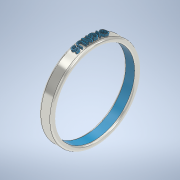
# Autodesk Inventor part: Repujado 3
Saved by Autodesk Inventor 2021 (Build 250183000, 183)
## iProperties
Created: 2021-01-13
Part Number: Repujado 3
Material: Genérico
Document SubType Name: Modeling
Designer: yosaf
Density: 1 g/cm^3
Appearance: Valor por defecto
Author: yosaf
Autodesk Inventor part; units mm, degrees
ref_plane "YZ Plane" through (0, 0, 0) normal (1, 0, 0) x (0, 1, 0)
ref_plane "XY Plane" through (0, 0, 0) normal (0, 0, 1) x (1, 0, 0)
sketch "Boceto1" plane through (0, 0, 0) normal (1, 0, 0) x (0, 1, 0)
  circle A0 centre (0, 0) radius 10
  dimension "d0" = 20
  constraints: 1 centre point, 1 coincident
  measures "d0" diameter of A0
extrude "Extrusión1" add sketch "Boceto1" along normal blind 3
sketch "Boceto2" plane through (3, 0, 0) normal (1, 0, 0) x (0, 0, -1)
  circle A0 centre (0, 0) radius 9
  dimension "d3" = 18
  constraints: 1 centre point, 1 coincident
  measures "d3" diameter of A0
extrude "Extrusión2" cut sketch "Boceto2" against normal blind 3
fillet "Empalme1" radius 0.5 4 edges at (3, -10, 0) (3, 0, 9) (0, -10, 0) (0, 0, 9)
ref_plane "Plano de trabajo1" through (0, 10, 0) normal (0, 1, 0) x (-1, 0, 0)
sketch "Boceto3" plane through (0, 10, 0) normal (0, 1, 0) x (-1, 0, 0)
  line L0 (-2.2914, -3.8707) -> (-2.2914, 3.8129) construction
  line L1 (-2.2914, 3.8129) -> (-0.4993, 3.8129) construction
  line L2 (-0.4993, 3.8129) -> (-0.4993, -3.8707) construction
  line L3 (-0.4993, -3.8707) -> (-2.2914, -3.8707) construction
  spline S0 degree 2 poles (-0.7379, -3.1328) (-0.7379, -3.2787) (-0.8363, -3.5254) (-0.9348, -3.6154) knots 0 0 0 1 2 2 2
  spline S1 degree 2 poles (-0.9348, -3.6154) (-1.032, -3.7053) (-1.3238, -3.8038) (-1.5134, -3.8038) knots 0 0 0 1 2 2 2
  spline S2 degree 2 poles (-1.5134, -3.8038) (-1.7018, -3.8038) (-1.9814, -3.7078) (-2.0847, -3.6166) knots 0 0 0 1 2 2 2
  spline S3 degree 2 poles (-2.0847, -3.6166) (-2.1856, -3.5267) (-2.2914, -3.2811) (-2.2914, -3.1292) knots 0 0 0 1 2 2 2
  spline S4 degree 2 poles (-2.2914, -3.1292) (-2.2914, -3.0538) (-2.2695, -2.9213) (-2.2525, -2.8654) knots 0 0 0 1 2 2 2
  spline S5 degree 2 poles (-2.2525, -2.8654) (-2.2367, -2.8168) (-2.1917, -2.7159) (-2.1649, -2.666) knots 0 0 0 1 2 2 2
  line L4 (-2.1649, -2.666) -> (-1.9243, -2.666)
  line L5 (-1.9243, -2.666) -> (-1.9243, -2.6818)
  spline S6 degree 2 poles (-1.9243, -2.6818) (-1.9486, -2.7086) (-2.0166, -2.7912) (-2.0495, -2.8508) knots 0 0 0 1 2 2 2
  spline S7 degree 2 poles (-2.0495, -2.8508) (-2.0811, -2.9079) (-2.1212, -3.0429) (-2.1212, -3.1304) knots 0 0 0 1 2 2 2
  spline S8 degree 2 poles (-2.1212, -3.1304) (-2.1212, -3.2264) (-2.0422, -3.3978) (-1.9668, -3.4622) knots 0 0 0 1 2 2 2
  spline S9 degree 2 poles (-1.9668, -3.4622) (-1.8902, -3.5254) (-1.6581, -3.5959) (-1.5134, -3.5959) knots 0 0 0 1 2 2 2
  spline S10 degree 2 poles (-1.5134, -3.5959) (-1.359, -3.5959) (-1.1366, -3.5218) (-1.06, -3.4574) knots 0 0 0 1 2 2 2
  spline S11 degree 2 poles (-1.06, -3.4574) (-0.9859, -3.3942) (-0.9105, -3.2252) (-0.9105, -3.1304) knots 0 0 0 1 2 2 2
  spline S12 degree 2 poles (-0.9105, -3.1304) (-0.9105, -3.0441) (-0.953, -2.897) (-0.9846, -2.8399) knots 0 0 0 1 2 2 2
  spline S13 degree 2 poles (-0.9846, -2.8399) (-1.0162, -2.7852) (-1.0819, -2.7037) (-1.105, -2.6806) knots 0 0 0 1 2 2 2
  line L6 (-1.105, -2.6806) -> (-1.105, -2.666)
  line L7 (-1.105, -2.666) -> (-0.8667, -2.666)
  spline S14 degree 2 poles (-0.8667, -2.666) (-0.8436, -2.7159) (-0.8011, -2.8034) (-0.7816, -2.8654) knots 0 0 0 1 2 2 2
  spline S15 degree 2 poles (-0.7816, -2.8654) (-0.7598, -2.931) (-0.7379, -3.0429) (-0.7379, -3.1328) knots 0 0 0 1 2 2 2
  line L8 (-2.2646, -1.4298) -> (-1.4283, -1.9367)
  line L9 (-1.4283, -1.9367) -> (-0.7646, -1.9367)
  line L10 (-0.7646, -1.9367) -> (-0.7646, -2.1361)
  line L11 (-0.7646, -2.1361) -> (-1.4077, -2.1361)
  line L12 (-1.4077, -2.1361) -> (-2.2646, -2.6429)
  line L13 (-2.2646, -2.6429) -> (-2.2646, -2.4217)
  line L14 (-2.2646, -2.4217) -> (-1.6046, -2.0352)
  line L15 (-1.6046, -2.0352) -> (-2.2646, -1.6413)
  line L16 (-2.2646, -1.6413) -> (-2.2646, -1.4298)
  spline S16 degree 2 poles (-0.7354, -0.6628) (-0.7354, -0.822) (-0.8327, -1.0858) (-0.9312, -1.1806) knots 0 0 0 1 2 2 2
  spline S17 degree 2 poles (-0.9312, -1.1806) (-1.0308, -1.2754) (-1.325, -1.3763) (-1.5158, -1.3763) knots 0 0 0 1 2 2 2
  spline S18 degree 2 poles (-1.5158, -1.3763) (-1.697, -1.3763) (-1.9838, -1.2742) (-2.0859, -1.1794) knots 0 0 0 1 2 2 2
  spline S19 degree 2 poles (-2.0859, -1.1794) (-2.1844, -1.0882) (-2.2914, -0.8208) (-2.2914, -0.6616) knots 0 0 0 1 2 2 2
  spline S20 degree 2 poles (-2.2914, -0.6616) (-2.2914, -0.585) (-2.2695, -0.4464) (-2.25, -0.3832) knots 0 0 0 1 2 2 2
  spline S21 degree 2 poles (-2.25, -0.3832) (-2.2354, -0.3322) (-2.182, -0.2082) (-2.1625, -0.1705) knots 0 0 0 1 2 2 2
  line L17 (-2.1625, -0.1705) -> (-1.9218, -0.1705)
  line L18 (-1.9218, -0.1705) -> (-1.9218, -0.1875)
  spline S22 degree 2 poles (-1.9218, -0.1875) (-1.9547, -0.2252) (-2.0142, -0.3042) (-2.0482, -0.3771) knots 0 0 0 1 2 2 2
  spline S23 degree 2 poles (-2.0482, -0.3771) (-2.0786, -0.4379) (-2.1188, -0.5947) (-2.1188, -0.6847) knots 0 0 0 1 2 2 2
  spline S24 degree 2 poles (-2.1188, -0.6847) (-2.1188, -0.901) (-1.793, -1.1685) (-1.5219, -1.1685) knots 0 0 0 1 2 2 2
  spline S25 degree 2 poles (-1.5219, -1.1685) (-1.3712, -1.1685) (-1.1451, -1.098) (-1.0673, -1.0311) knots 0 0 0 1 2 2 2
  spline S26 degree 2 poles (-1.0673, -1.0311) (-0.9895, -0.9667) (-0.9081, -0.7844) (-0.9081, -0.6701) knots 0 0 0 1 2 2 2
  spline S27 degree 2 poles (-0.9081, -0.6701) (-0.9081, -0.5862) (-0.9324, -0.4185) (-0.9567, -0.3613) knots 0 0 0 1 2 2 2
  line L19 (-0.9567, -0.3613) -> (-1.3444, -0.3613)
  line L20 (-1.3444, -0.3613) -> (-1.3444, -0.709)
  line L21 (-1.3444, -0.709) -> (-1.5195, -0.709)
  line L22 (-1.5195, -0.709) -> (-1.5195, -0.1644)
  line L23 (-1.5195, -0.1644) -> (-0.8643, -0.1644)
  spline S28 degree 2 poles (-0.8643, -0.1644) (-0.8473, -0.2021) (-0.795, -0.331) (-0.7792, -0.3857) knots 0 0 0 1 2 2 2
  spline S29 degree 2 poles (-0.7792, -0.3857) (-0.7573, -0.4598) (-0.7354, -0.5789) (-0.7354, -0.6628) knots 0 0 0 1 2 2 2
  line L24 (-0.7646, 1.1593) -> (-0.7646, 0.9357)
  line L25 (-0.7646, 0.9357) -> (-2.058, 0.272)
  line L26 (-2.058, 0.272) -> (-0.7646, 0.272)
  line L27 (-0.7646, 0.272) -> (-0.7646, 0.086)
  line L28 (-0.7646, 0.086) -> (-2.2646, 0.086)
  line L29 (-2.2646, 0.086) -> (-2.2646, 0.3692)
  line L30 (-2.2646, 0.3692) -> (-1.077, 0.9733)
  line L31 (-1.077, 0.9733) -> (-2.2646, 0.9733)
  line L32 (-2.2646, 0.9733) -> (-2.2646, 1.1593)
  line L33 (-2.2646, 1.1593) -> (-0.7646, 1.1593)
  spline S30 degree 2 poles (-0.733, 1.9871) (-0.733, 1.8546) (-0.8023, 1.6577) (-0.8716, 1.5884) knots 0 0 0 1 2 2 2
  spline S31 degree 2 poles (-0.8716, 1.5884) (-0.9494, 1.5094) (-1.1682, 1.445) (-1.3286, 1.445) knots 0 0 0 1 2 2 2
  line L34 (-1.3286, 1.445) -> (-2.2646, 1.445)
  line L35 (-2.2646, 1.445) -> (-2.2646, 1.6443)
  line L36 (-2.2646, 1.6443) -> (-1.3286, 1.6443)
  spline S32 degree 2 poles (-1.3286, 1.6443) (-1.2241, 1.6443) (-1.0831, 1.6711) (-1.026, 1.7088) knots 0 0 0 1 2 2 2
  spline S33 degree 2 poles (-1.026, 1.7088) (-0.9652, 1.7489) (-0.9032, 1.8874) (-0.9032, 1.9871) knots 0 0 0 1 2 2 2
  spline S34 degree 2 poles (-0.9032, 1.9871) (-0.9032, 2.0807) (-0.9652, 2.2266) (-1.026, 2.2667) knots 0 0 0 1 2 2 2
  spline S35 degree 2 poles (-1.026, 2.2667) (-1.0831, 2.3044) (-1.2229, 2.3311) (-1.3238, 2.3311) knots 0 0 0 1 2 2 2
  line L37 (-1.3238, 2.3311) -> (-2.2646, 2.3311)
  line L38 (-2.2646, 2.3311) -> (-2.2646, 2.5305)
  line L39 (-2.2646, 2.5305) -> (-1.3286, 2.5305)
  spline S36 degree 2 poles (-1.3286, 2.5305) (-1.1718, 2.5305) (-0.9482, 2.4673) (-0.8716, 2.387) knots 0 0 0 1 2 2 2
  spline S37 degree 2 poles (-0.8716, 2.387) (-0.8011, 2.3153) (-0.733, 2.1257) (-0.733, 1.9871) knots 0 0 0 1 2 2 2
  spline S38 degree 2 poles (-0.7379, 3.2343) (-0.7379, 3.0714) (-0.8059, 2.8429) (-0.8546, 2.742) knots 0 0 0 1 2 2 2
  line L40 (-0.8546, 2.742) -> (-1.105, 2.742)
  line L41 (-1.105, 2.742) -> (-1.105, 2.7566)
  spline S39 degree 2 poles (-1.105, 2.7566) (-1.0126, 2.855) (-0.9105, 3.1042) (-0.9105, 3.2197) knots 0 0 0 1 2 2 2
  spline S40 degree 2 poles (-0.9105, 3.2197) (-0.9105, 3.385) (-1.0478, 3.554) (-1.1609, 3.554) knots 0 0 0 1 2 2 2
  spline S41 degree 2 poles (-1.1609, 3.554) (-1.2508, 3.554) (-1.3627, 3.4652) (-1.3906, 3.3692) knots 0 0 0 1 2 2 2
  spline S42 degree 2 poles (-1.3906, 3.3692) (-1.4101, 3.2999) (-1.4368, 3.1844) (-1.4587, 3.0981) knots 0 0 0 1 2 2 2
  spline S43 degree 2 poles (-1.4587, 3.0981) (-1.4794, 3.0203) (-1.5414, 2.8976) (-1.5912, 2.8502) knots 0 0 0 1 2 2 2
  spline S44 degree 2 poles (-1.5912, 2.8502) (-1.641, 2.804) (-1.7747, 2.7529) (-1.8623, 2.7529) knots 0 0 0 1 2 2 2
  spline S45 degree 2 poles (-1.8623, 2.7529) (-2.0446, 2.7529) (-2.2914, 3.0374) (-2.2914, 3.2574) knots 0 0 0 1 2 2 2
  spline S46 degree 2 poles (-2.2914, 3.2574) (-2.2914, 3.3838) (-2.2415, 3.6075) (-2.1941, 3.7035) knots 0 0 0 1 2 2 2
  line L42 (-2.1941, 3.7035) -> (-1.9559, 3.7035)
  line L43 (-1.9559, 3.7035) -> (-1.9559, 3.6889)
  spline S47 degree 2 poles (-1.9559, 3.6889) (-2.0215, 3.6172) (-2.1188, 3.3935) (-2.1188, 3.2708) knots 0 0 0 1 2 2 2
  spline S48 degree 2 poles (-2.1188, 3.2708) (-2.1188, 3.1322) (-1.9887, 2.9608) (-1.8829, 2.9608) knots 0 0 0 1 2 2 2
  spline S49 degree 2 poles (-1.8829, 2.9608) (-1.7881, 2.9608) (-1.6751, 3.0617) (-1.6495, 3.1565) knots 0 0 0 1 2 2 2
  spline S50 degree 2 poles (-1.6495, 3.1565) (-1.6325, 3.2197) (-1.5888, 3.4032) (-1.5705, 3.464) knots 0 0 0 1 2 2 2
  spline S51 degree 2 poles (-1.5705, 3.464) (-1.5231, 3.6184) (-1.3323, 3.7618) (-1.1925, 3.7618) knots 0 0 0 1 2 2 2
  spline S52 degree 2 poles (-1.1925, 3.7618) (-1.1038, 3.7618) (-0.9336, 3.6901) (-0.874, 3.6257) knots 0 0 0 1 2 2 2
  spline S53 degree 2 poles (-0.874, 3.6257) (-0.8084, 3.554) (-0.7379, 3.3716) (-0.7379, 3.2343) knots 0 0 0 1 2 2 2
  point P0 (0, 0)
  constraints: 2 other
emboss "Repujado1" sketch "Boceto3" operation add depth 0.5 direction (0, -1, 0) wrap yes faces at (1.8334, 9.9676, -0.8047)
